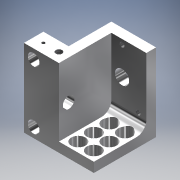
# Autodesk Inventor part: Probenkammer Halter Plus-Seite
Saved by Autodesk Inventor 2017 (Build 210142000, 142)
## iProperties
Part Number: Probenkammer Halter Plus-Seite
Material: Aluminium 6061
Document SubType Name: Modeling
Designer: David Merges
Density: 2.7 g/cm^3
Appearance: Aluminium - flach
Author: David Merges
Autodesk Inventor part; units mm, degrees
ref_plane "YZ Plane" through (0, 0, 0) normal (1, 0, 0) x (0, 1, 0)
ref_plane "XZ Plane" through (0, 0, 0) normal (0, 1, 0) x (-1, 0, 0)
ref_plane "XY Plane" through (0, 0, 0) normal (0, 0, 1) x (1, 0, 0)
sketch "Skizze1" plane through (0, 0, 0) normal (0, 1, 0) x (-1, 0, 0)
  line L0 (5, 20) -> (-13, 20)
  line L1 (-13, 20) -> (-13, -20)
  line L2 (-13, -20) -> (5, -20)
  line L3 (5, -20) -> (5, 20)
  line L4 (0, 15) -> (0, -15) construction
  line L5 (5, 0) -> (0, 0) construction
  circle A0 centre (0, -15) radius 3
  circle A1 centre (0, 15) radius 3
  dimension "d0" = 30
  dimension "d1" = 40
  dimension "d2" = 6
  dimension "d5" = 5
  dimension "d6" = 13
  constraints: 12 end point, 3 coincident, 2 centre point, 2 midpoint, 2 parallel, 2 perpendicular, 1 equal radius, 1 horizontal, 1 vertical
  measures "d0" distance of L4.start L4.end
  measures "d1" distance of L2.end L0.start
  measures "d2" diameter of A0
  measures "d5" distance between parallel lines of L3 L4
  measures "d6" distance between parallel lines of L4 L1
extrude "Extrusion1" add sketch "Skizze1" along normal mid plane 10
sketch "Skizze2" plane through (13, -5, -20) normal (1, 0, 0) x (0, 0, -1)
  circle A0 centre (-20, 5) radius 3
  point P0 (-20, 5)
  dimension "d7" = 6
  constraints: 1 centre point, 1 coincident
  measures "d7" diameter of A0
extrude "Extrusion2" cut sketch "Skizze2" against normal through all
sketch "Skizze3" plane through (-5, 5, 20) normal (0, 0, 1) x (1, 0, 0)
  line L0 (18, -10) -> (18, 0) projected
  line L1 (18, -5) -> (13, -5) construction
  point P0 (5, -5)
  dimension "d10" = 5
  constraints: 2 end point, 1 coincident, 1 midpoint, 1 perpendicular
  measures "d10" distance of L1.start L1.end
hole "Bohrung1" at (8, 0, 20) direction (0, 0, -1) diameter 3.242 end up to surface thread size "M4x0.7" class "6H" standard "ISO Metric profile"
sketch "Skizze4" plane through (-5, 5, 20) normal (0, 0, 1) x (1, 0, 0)
  point P0 (5, -5)
hole "Bohrung2" at (0, 0, 20) direction (0, 0, -1) diameter 1.567 depth 6.3 tip angle 118 thread size "M2x0.4" class "6H" standard "ISO Metric profile"
mirror "Spiegeln2" about plane through (0, 0, 0) normal (0, 0, 1) of "Bohrung2"
sketch "Skizze5" plane through (13, -5, -20) normal (1, 0, 0) x (0, 0, -1)
  circle A0 centre (-20, 5) radius 3 projected
  line L0 (0, 0) -> (0, 10) projected
  line L1 (-40, 10) -> (0, 10) projected
  line L2 (-40, 0) -> (-40, 10) projected
  line L3 (0, 0) -> (-40, 0) projected
  line L4 (-40, 10) -> (0, 10)
  line L5 (0, 10) -> (0, 26)
  line L6 (0, 26) -> (-40, 26)
  line L7 (-40, 26) -> (-40, 10)
  point P0 (-20, 5)
  dimension "d25" = 16
  constraints: 8 end point, 2 parallel, 1 horizontal, 1 perpendicular
  measures "d25" distance of L4.end L5.end
extrude "Extrusion3" add sketch "Skizze5" against normal blind 5 contours L1 L7 L6 L5
sketch "Skizze8" plane through (13, -5, 20) normal (1, 0, 0) x (0, 0, -1)
  circle A0 centre (20, 5) radius 3 projected
  line L0 (40, 0) -> (40, 26) projected
  line L1 (40, 26) -> (0, 26) projected
  line L2 (0, 0) -> (0, 26) projected
  line L3 (40, 0) -> (0, 0) projected
  line L4 (40, 0) -> (35, 0)
  line L5 (35, 0) -> (35, 26)
  line L6 (35, 26) -> (40, 26)
  line L7 (40, 26) -> (40, 0)
  point P0 (20, 5)
  dimension "d40" = 5
  constraints: 8 end point, 2 parallel, 1 horizontal, 1 perpendicular, 1 point on line
  measures "d40" distance between parallel lines of L5 L0
extrude "Extrusion5" add sketch "Skizze8" along normal blind 18 contours L3 L5 L1 L0
sketch "Skizze9" plane through (13, -5, -15) normal (0, 0, 1) x (1, 0, 0)
  line L0 (0, 0) -> (0, 26) projected
  line L1 (0, 0) -> (18, 0) projected
  line L2 (18, 26) -> (18, 0) projected
  line L3 (0, 26) -> (18, 26) projected
  line L4 (0, 0) -> (0, 26) construction
  line L5 (0, 13) -> (5, 13) construction
  line L6 (13, 5) -> (5, 5) construction
  line L7 (5, 5) -> (5, 13) construction
  line L8 (5, 13) -> (13, 13) construction
  line L9 (13, 13) -> (13, 5) construction
  line L10 (5, 13) -> (13, 13) construction
  line L11 (13, 13) -> (13, 21) construction
  line L12 (13, 21) -> (5, 21) construction
  line L13 (5, 21) -> (5, 13) construction
  point P0 (-13, 5)
  dimension "d43" = 5
  dimension "d44" = 8
  constraints: 18 end point, 6 coincident, 4 parallel, 4 perpendicular, 3 horizontal, 1 midpoint, 1 point on line
  measures "d43" distance of L5.start L5.end
  measures "d44" distance of L8.end L6.start
hole "Bohrung4" at (18, 0, -15) at (18, 8, -15) at (18, 16, -15) at (26, 16, -15) at (26, 8, -15) at (26, 0, -15) direction (0, 0, -1) diameter 7.3 end through all
sketch "Skizze10" plane through (8, 21, 20) normal (0, 1, 0) x (1, 0, 0)
  line L0 (0, 40) -> (23, 40) projected
  line L1 (0, 0) -> (0, 40) projected
  line L2 (5, 0) -> (0, 0) projected
  line L3 (5, 35) -> (5, 0) projected
  line L4 (5, 35) -> (23, 35) projected
  line L5 (23, 40) -> (23, 35) projected
  point P0 (-8, 20)
extrude "Extrusion6" add sketch "Skizze10" along normal blind 6
sketch "Skizze11" plane through (13, -5, 20) normal (1, 0, 0) x (0, 0, -1)
  line L0 (35, 0) -> (35, 32) projected
  line L1 (0, 32) -> (35, 32) projected
  line L2 (0, 0) -> (0, 32) projected
  line L3 (35, 0) -> (0, 0) projected
  circle A0 centre (20, 5) radius 3 projected
  line L4 (0, 10) -> (0, 32) projected
  line L5 (35, 0) -> (35, 32) projected
  line L6 (0, 32) -> (35, 32)
  line L7 (35, 32) -> (35, 27)
  line L8 (35, 27) -> (0, 27)
  line L9 (0, 27) -> (0, 32)
  point P0 (20, 5)
  dimension "d54" = 5
  constraints: 8 end point, 2 parallel, 1 horizontal, 1 perpendicular, 1 point on line
  measures "d54" distance between parallel lines of L6 L8
extrude "Extrusion7" add sketch "Skizze11" along normal up to surface (18 mm away) contours L8 L2 L1 L0
sketch "Skizze12" plane through (8, 27, 20) normal (0, 1, 0) x (1, 0, 0)
  line L0 (23, 40) -> (0, 40) projected
  line L1 (0, 40) -> (0, 0) projected
  line L2 (0, 0) -> (23, 0) projected
  line L3 (23, 0) -> (23, 40) projected
  line L4 (0, 0) -> (-3, 0)
  line L5 (-3, 0) -> (-3, 40)
  line L6 (-3, 40) -> (0, 40)
  line L7 (0, 40) -> (0, 0)
  line L8 (23, 40) -> (0, 40) projected
  line L9 (-3, 0) -> (10.5, 0) construction
  line L10 (10.5, 0) -> (10.5, 17) construction
  line L11 (10.5, 17) -> (-3, 17) construction
  line L12 (-3, 17) -> (-3, 0) construction
  point P0 (-8, 20)
  dimension "d57" = 3
  dimension "d58" = 13.5
  dimension "d59" = 17
  constraints: 16 end point, 4 parallel, 2 horizontal, 2 perpendicular, 1 coincident, 1 collinear
  measures "d57" distance between parallel lines of L1 L5
  measures "d58" distance between parallel lines of L5 L10
  measures "d59" distance of L9.end L10.end
hole "Bohrung5" at (18.5, 27, 3) direction (0, -1, 0) diameter 7.3 end through all
sketch "Skizze13" plane through (8, 27, 20) normal (0, 1, 0) x (1, 0, 0)
  circle A0 centre (10.5, 17) radius 3.65 projected
  line L0 (23, 40) -> (0, 40) projected
  line L1 (0, 40) -> (0, 0) projected
  line L2 (0, 0) -> (23, 0) projected
  line L3 (23, 0) -> (23, 40) projected
  circle A1 centre (10.5, 17) radius 3.65 construction
  line L4 (10.5, 17) -> (10.5, 2.6) construction
  line L5 (10.5, 17) -> (18.7595, 28.7958) construction
  line L6 (18.7595, 28.7958) -> (10.5, 17) construction
  line L7 (10.5, 17) -> (2.2405, 28.7958) construction
  point P0 (-8, 20)
  dimension "d75" = 14.4
  dimension "d76" = 70
  dimension "d77" = 35
  constraints: 8 end point, 3 coincident, 2 equal length, 1 vertical
  measures "d75" distance of L4.start L4.end
  measures "d76" angle of L5 L7
  measures "d77" angle of L6 L4
hole "Bohrung6" at (18.5, 27, 17.4) at (26.7595, 27, -8.7958) at (10.2405, 27, -8.7958) direction (0, -1, 0) diameter 2.459 depth 8.8 tip angle 118 thread size "M3x0.5" class "6H" standard "ISO Metric profile"
fillet "Rundung1" radius 5 1 edges at (22, 22, -15)
equation "\"d77\" = 0.5 * d76"
